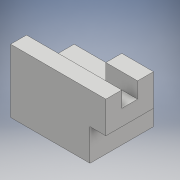
# Autodesk Inventor part: 11
Saved by Autodesk Inventor 2017 (Build 210142000, 142)
## iProperties
Part Number: 11
Material: 一般
Document SubType Name: Modeling
Designer: Brian
Density: 1 g/cm^3
Appearance: 預設
Author: Brian
Autodesk Inventor part; units mm, degrees
ref_plane "YZ Plane" through (0, 0, 0) normal (1, 0, 0) x (0, 1, 0)
ref_plane "XZ Plane" through (0, 0, 0) normal (0, 1, 0) x (-1, 0, 0)
ref_plane "XY Plane" through (0, 0, 0) normal (0, 0, 1) x (1, 0, 0)
sketch "草圖1" plane through (0, 0, 0) normal (0, 1, 0) x (-1, 0, 0)
  line L0 (0, 0) -> (-60, 0)
  line L1 (-60, 0) -> (-60, -20)
  line L2 (-60, -20) -> (0, -20)
  line L3 (0, -20) -> (0, 0)
  dimension "d0" = 20
  dimension "d1" = 60
  constraints: 8 end point, 2 parallel, 1 horizontal, 1 perpendicular
  measures "d0" distance of L2.end L0.start
  measures "d1" distance of L1.end L2.end
extrude "擠出1" add sketch "草圖1" along normal blind 10
sketch "草圖2" plane through (60, 0, -20) normal (0, 0, -1) x (-1, 0, 0)
  line L0 (60, 0) -> (0, 0) projected
  line L1 (60, 0) -> (10, 0)
  line L2 (10, 0) -> (10, 40)
  line L3 (10, 40) -> (60, 40)
  line L4 (60, 40) -> (60, 0)
  dimension "d4" = 50
  dimension "d5" = 40
  constraints: 8 end point, 2 parallel, 1 horizontal, 1 perpendicular
  measures "d4" distance of L2.end L3.end
  measures "d5" distance of L1.end L2.end
extrude "擠出2" add sketch "草圖2" along normal blind 20
sketch "草圖3" plane through (60, 0, 0) normal (1, 0, 0) x (0, 0, -1)
  line L0 (20, 10) -> (20, 40) projected
  line L1 (20, 10) -> (10, 10)
  line L2 (10, 10) -> (10, 20)
  line L3 (10, 20) -> (20, 20)
  line L4 (20, 20) -> (20, 10)
  line L5 (20, 20) -> (0, 20)
  line L6 (0, 20) -> (0, 30)
  line L7 (0, 30) -> (20, 30)
  line L8 (20, 30) -> (20, 20)
  point P0 (0, 0)
  dimension "d8" = 20
  dimension "d9" = 10
  dimension "d10" = 10
  dimension "d11" = 10
  constraints: 16 end point, 4 parallel, 2 horizontal, 2 perpendicular
  measures "d8" distance of L6.end L7.end
  measures "d9" distance between parallel lines of L0 L2
  measures "d10" distance of L5.end L6.end
  measures "d11" distance of L1.end L2.end
extrude "擠出3" add sketch "草圖3" against normal blind 20
